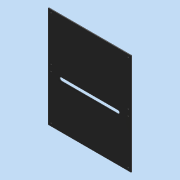
# Autodesk Inventor part: FrameTop
Saved by Autodesk Inventor 2016 (Build 200138000, 138)
## iProperties
Created: 2016-08-20
Part Number: FrameTop
Material: Dibond
Document SubType Name: Modeling
Designer: Sam
Density: 1 g/cm^3
Appearance: Generic
Author: Sam
Autodesk Inventor part; units mm, degrees
ref_plane "YZ Plane" through (0, 0, 0) normal (1, 0, 0) x (0, 1, 0)
ref_plane "XZ Plane" through (0, 0, 0) normal (0, 1, 0) x (-1, 0, 0)
ref_plane "XY Plane" through (0, 0, 0) normal (0, 0, 1) x (1, 0, 0)
sketch "Sketch1" plane through (0, 0, 0) normal (0, 1, 0) x (-1, 0, 0)
  line L0 (0, 0) -> (360, 0)
  line L1 (360, 0) -> (360, -440)
  line L2 (360, -440) -> (0, -440)
  line L3 (0, -440) -> (0, 0)
  dimension "d0" = 360
  dimension "d1" = 440
  constraints: 8 end point, 2 parallel, 1 horizontal, 1 perpendicular
  measures "d0" distance of L1.end L2.end
  measures "d1" distance of L0.end L1.end
extrude "Extrusion1" add sketch "Sketch1" along normal blind 3
hole "Hole1" at (-12, 3, -12) direction (0, -1, 0) diameter 4 end through all
hole "Hole2" at (-348, 3, -12) direction (0, -1, 0) diameter 4 end through all
hole "Hole3" at (-348, 3, -428) direction (0, -1, 0) diameter 4 end through all
hole "Hole4" at (-12, 3, -428) direction (0, -1, 0) diameter 4 end through all
hole "Hole5" at (-12, 3, -206.5) direction (0, -1, 0) diameter 4 end through all
hole "Hole6" at (-12, 3, -233.5) direction (0, -1, 0) diameter 4 end through all
hole "Hole7" at (-348, 3, -206.5) direction (0, -1, 0) diameter 4 end through all
hole "Hole8" at (-348, 3, -233.5) direction (0, -1, 0) diameter 4 end through all
sketch "Sketch2" plane through (0, 3, 0) normal (0, 1, 0) x (1, 0, 0)
  line L0 (-360, 440) -> (-360, 0) projected
  line L1 (-360, 220) -> (0, 220)
  line L2 (0, 440) -> (0, 0) projected
  line L3 (-310, 240) -> (-50, 240) construction
  line L4 (-303, 233) -> (-57, 233)
  line L5 (-57, 247) -> (-303, 247)
  arc A0 (-303, 247) -> (-303, 233) centre (-303, 240) ccw
  arc A1 (-57, 233) -> (-57, 247) centre (-57, 240) ccw
  point P0 (-180, 240)
  constraints: 10 end point, 6 point on circle, 4 tangent, 3 midpoint, 2 centre point, 2 point on line, 1 parallel, 1 perpendicular
extrude "Extrusion2" cut sketch "Sketch2" against normal blind 3
fillet "Fillet1" radius 2 4 edges at (-50, 3, -240) (-180, 3, -233) (-310, 3, -240) (-180, 3, -247)
body "Solid1"
